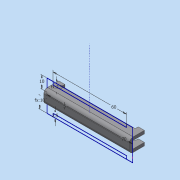
# Autodesk Inventor part: 0 零件
Saved by Autodesk Inventor 2020 (Build 240168000, 168)
## iProperties
Created: 2020-11-03
Part Number: 0 零件
Material: 一般
Document SubType Name: Modeling
Designer: p2013
Density: 1 g/cm^3
Appearance: 預設
Author: p2013
Autodesk Inventor part; units mm, degrees
ref_plane "YZ Plane" through (0, 0, 0) normal (1, 0, 0) x (0, 1, 0)
ref_plane "XZ Plane" through (0, 0, 0) normal (0, 1, 0) x (-1, 0, 0)
ref_plane "XY Plane" through (0, 0, 0) normal (0, 0, 1) x (1, 0, 0)
sketch "草圖1" plane through (0, 0, 0) normal (0, 0, 1) x (1, 0, 0)
  line L0 (0, 0) -> (0, 51.6107) construction
  line L1 (-35, -5) -> (35, -5)
  line L2 (35, -5) -> (35, -15)
  line L3 (35, -15) -> (-35, -15)
  line L4 (-35, -15) -> (-35, -5)
  line L5 (-35, -5) -> (35, -5)
  line L6 (35, -5) -> (35, 0)
  line L7 (35, 0) -> (-35, 0)
  line L8 (-35, 0) -> (-35, -5)
  line L9 (35, -12) -> (35, 0)
  line L10 (-35, -12) -> (-35, 0)
  line L11 (-35, 0) -> (35, 0)
  line L12 (35, 0) -> (35, 10)
  line L13 (35, 10) -> (-35, 10)
  line L14 (-35, 10) -> (-35, 0)
  line L15 (-30, 10) -> (30, 10)
  line L16 (30, 10) -> (30, 7.5)
  line L17 (30, 7.5) -> (-30, 7.5)
  line L18 (-30, 7.5) -> (-30, 10)
  line L19 (-30, -15) -> (30, -15)
  line L20 (30, -15) -> (30, -12.5)
  line L21 (30, -12.5) -> (-30, -12.5)
  line L22 (-30, -12.5) -> (-30, -15)
  line L23 (-20, 4.3118) -> (-17, 4.3118)
  line L24 (-17, 4.3118) -> (-17, -10)
  line L25 (-17, -10) -> (-20, -10)
  line L26 (-20, -10) -> (-20, 4.3118)
  line L27 (20, 4.3118) -> (17, 4.3118)
  line L28 (17, 4.3118) -> (17, -10)
  line L29 (17, -10) -> (20, -10)
  line L30 (20, -10) -> (20, 4.3118)
  point P0 (30, -15)
  point P1 (35, 0)
  dimension "d2" = 70
  dimension "d3" = 5
  dimension "d13" = 2.5
  dimension "d14" = 2.5
  dimension "d15" = 10
  dimension "d16" = 10
  dimension "d17" = 60
  dimension "d18" = 3
  dimension "d19" = 40
  constraints: 62 end point, 12 parallel, 6 horizontal, 6 perpendicular, 4 symmetric about line, 3 point on line, 2 collinear, 1 midpoint, 1 vertical, 3 other
  measures "d2" distance between parallel lines of L6 L8
  measures "d3" distance between parallel lines of L7 L1
  measures "d13" distance between parallel lines of L3 L21
  measures "d14" distance between parallel lines of L13 L17
  measures "d15" distance between parallel lines of L7 L13
  measures "d16" distance between parallel lines of L3 L1
  measures "d17" distance of L16.end L17.end
  measures "d18" distance between parallel lines of L24 L26
  measures "d19" distance between parallel lines of L30 L26
extrude "擠出1" add sketch "草圖1" along normal blind 2.5 contours L8 L7 L26 L1 | L1 L26 L25 L24 L28 L29 L30 L2 L3 L20 L21 L22 L4 | L14 L13 L18 L17 L16 L12 L7 L30 L27 L28 L24 L23 L26 | L24 L7 L28 L1 | L30 L7 L6 L1
bend part "折彎零件1" radius 0.5 angle 90 line through (-35, 0, 0) along (1, 0, 0) centre toward (0, 0, -1) moving side (0, 1, 0) both sides no
bend part "折彎零件3" radius 0.5 angle 90 line through (-35, -5, 0) along (1, 0, 0) centre toward (0, 0, -1) moving side (0, -1, 0) both sides no
equation "\"d14\" = d13"
equation "\"d16\" = d15"
